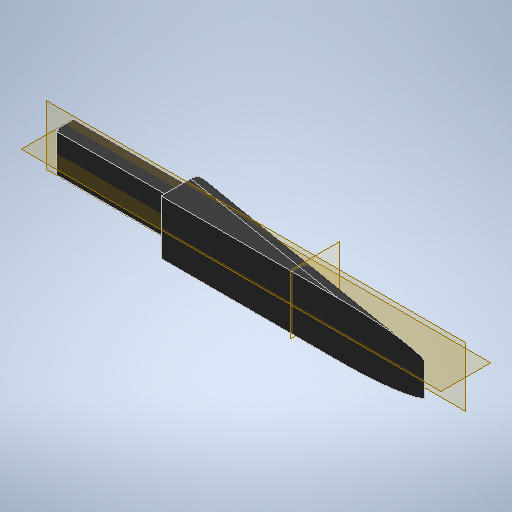
# Autodesk Inventor part: BracoRobotico_0003_002
Saved by Autodesk Inventor 2025.2 (Build 292293000, 293)
## iProperties
Created: 2025-05-28
Part Number: BracoRobotico_0003_002
Material: Rubber
Document SubType Name: Modeling
Designer: I
Density: 0.93 g/cm^3
Appearance: Rubber - Black
Author: I
Autodesk Inventor part; units mm, degrees
sketch "Sketch1" plane through (0, 0, 0) normal (0, 0, 1) x (1, 0, 0)
  line L0 (-43.75, -9) -> (43.75, -9)
  line L1 (43.75, -9) -> (43.75, 9)
  line L2 (43.75, 9) -> (-43.75, 9)
  line L3 (-43.75, 9) -> (-43.75, -9)
  line L4 (-43.75, -9) -> (43.75, 9) construction
  line L5 (43.75, -9) -> (-43.75, 9) construction
  point P0 (0, 0)
  dimension "d0" = 87.5
  dimension "d1" = 18
  constraints: 12 end point, 3 midpoint, 1 horizontal, 1 vertical
  measures "d0" distance of L1.end L2.end
  measures "d1" distance of L0.end L1.end
extrude "Extrusion1" add sketch "Sketch1" along normal mid plane 15
sketch "Sketch3" plane through (-43.75, 9, 7.5) normal (0, 1, 0) x (1, 0, 0)
  line L0 (0, 15) -> (87.5, 0.25)
  line L1 (87.5, 15) -> (87.5, 0) construction
  line L2 (87.5, 0.25) -> (87.5, 15)
  line L3 (87.5, 15) -> (0, 15)
  point P0 (43.75, 7.5)
  point P1 (87.5, 7.625)
  dimension "d5" = 0.25
  constraints: 6 end point, 2 point on line, 1 coincident, 1 midpoint
  measures "d5" distance of L1.end L0.end
extrude "Extrusion2" cut sketch "Sketch3" along normal through all both and the other way through all
sketch "Sketch5" plane through (-43.75, -9, 7.5) normal (-1, 0, 0) x (0, 0, 1)
  line L0 (-3.95, 2.75) -> (-10.3, 2.75)
  line L1 (-10.3, 2.75) -> (-10.3, 15.25)
  line L2 (-10.3, 15.25) -> (-3.95, 15.25)
  line L3 (-3.95, 15.25) -> (-3.95, 2.75)
  line L4 (-3.95, 2.75) -> (-10.3, 15.25) construction
  line L5 (-10.3, 2.75) -> (-3.95, 15.25) construction
  line L6 (0, 18) -> (0, 0) construction
  line L7 (-15, 0) -> (-15, 18) construction
  point P0 (-7.5, 9)
  point P1 (-7.125, 9)
  dimension "d14" = 12.5
  dimension "d28" = 3.95
  dimension "d29" = 4.7
  constraints: 12 end point, 2 midpoint, 1 horizontal, 1 horizontal alignment, 1 perpendicular
  measures "d14" distance of L2.end L0.start
  measures "d28" distance between parallel lines of L3 L6
  measures "d29" distance between parallel lines of L7 L1
extrude "Extrusion4" add sketch "Sketch5" along normal blind 38.75
sketch "Sketch7" plane through (0, 0, -2.8) normal (0, 0, 1) x (1, 0, 0)
  line L0 (-82.5, 6.25) -> (-82.5, -6.25) construction
  circle A0 centre (-131.7, 0) radius 49
  line L1 (43.75, -9) -> (43.75, 9) projected
  line L2 (-82.5, -6.25) -> (-83.1002, -6.25)
  line L3 (-82.5, 6.25) -> (-83.1002, 6.25)
  line L4 (-82.5, -6.25) -> (-82.5, 6.25)
  point P0 (0, 0)
  point P1 (43.75, 0)
  point P2 (-82.5, 0)
  dimension "d23" = 98
  dimension "d24" = 175.45
  constraints: 6 end point, 3 midpoint, 2 horizontal, 2 point on circle, 1 centre point, 1 horizontal alignment
  measures "d23" diameter of A0
  measures "d24" distance of point (43.75, 0) A0.centre
extrude "Extrusion5" add sketch "Sketch7" along normal blind 5.65 contours A0 L3 L4 L2
fillet "Fillet2" radius 5 2 edges at (0, 9, -0.125) (0, -9, -0.125)
equation "\"d25\" = d15"
equation "\"d15\" = 5.65"
body "Solid1"
